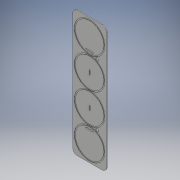
# Autodesk Inventor part: Cewki_840
Saved by Autodesk Inventor 2017 (Build 210142000, 142)
## iProperties
Created: 2019-10-27
Part Number: Cewki_840
Material: Ogólny
Document SubType Name: Modeling
Designer: patry
Density: 1 g/cm^3
Appearance: Domyślna
Author: patry
Autodesk Inventor part; units mm, degrees
ref_plane "YZ Plane" through (0, 0, 0) normal (1, 0, 0) x (0, 1, 0)
ref_plane "XZ Plane" through (0, 0, 0) normal (0, 1, 0) x (-1, 0, 0)
ref_plane "XY Plane" through (0, 0, 0) normal (0, 0, 1) x (1, 0, 0)
sketch "Szkic1" plane through (0, 0, 0) normal (0, 1, 0) x (-1, 0, 0)
  line L0 (-112.5, 420) -> (112.5, 420)
  line L1 (112.5, 420) -> (112.5, 262)
  line L2 (112.5, -420) -> (-112.5, -420)
  line L3 (-112.5, -420) -> (-112.5, 27)
  line L4 (-112.5, 420) -> (112.5, -420) construction
  line L5 (112.5, 420) -> (-112.5, -420) construction
  circle A0 centre (0, -307.5) radius 102.5
  circle A1 centre (0, -307.5) radius 95
  circle A2 centre (0, -102.5) radius 102.5
  circle A3 centre (0, -102.5) radius 95
  circle A4 centre (0, 102.5) radius 102.5
  circle A5 centre (0, 102.5) radius 95
  circle A6 centre (0, 307.5) radius 102.5
  circle A7 centre (0, 307.5) radius 95
  line L6 (-112.5, 27) -> (-112.5, 420)
  line L7 (0, 420) -> (0, -420) construction
  line L8 (112.5, 262) -> (112.5, 257)
  line L9 (112.5, 257) -> (112.5, -193)
  line L10 (112.5, -197.6604) -> (112.5, -420)
  line L11 (112.5, -193) -> (112.5, -197.6604)
  line L12 (-182, -225) -> (183, -225) construction
  line L13 (-175, 225) -> (225, 225) construction
  line L14 (-221, -230.5) -> (174, -230.5) construction
  line L15 (-175, 230.5) -> (202.5, 230.5) construction
  line L16 (23, 225) -> (-23, 225)
  line L17 (-25, 227) -> (-25, 228.5)
  line L18 (-23, 230.5) -> (23, 230.5)
  line L19 (25, 228.5) -> (25, 227)
  line L20 (-226, 0) -> (183, 0) construction
  arc A8 (23, 225) -> (25, 227) centre (23, 227) ccw
  arc A9 (25, 228.5) -> (23, 230.5) centre (23, 228.5) ccw
  arc A10 (-25, 227) -> (-23, 225) centre (-23, 227) ccw
  arc A11 (-23, 230.5) -> (-25, 228.5) centre (-23, 228.5) ccw
  line L21 (23, -225) -> (-23, -225)
  line L22 (-25, -227) -> (-25, -228.5)
  line L23 (-23, -230.5) -> (23, -230.5)
  line L24 (25, -228.5) -> (25, -227)
  arc A12 (25, -227) -> (23, -225) centre (23, -227) ccw
  arc A13 (23, -230.5) -> (25, -228.5) centre (23, -228.5) ccw
  arc A14 (-23, -225) -> (-25, -227) centre (-23, -227) ccw
  arc A15 (-25, -228.5) -> (-23, -230.5) centre (-23, -228.5) ccw
  line L25 (0, -212.5) -> (0, 284.5) construction
  line L26 (-55, -249) -> (-55, 249) construction
  line L27 (-0.75, -87.5) -> (0.75, -87.5)
  line L28 (2.75, -89.5) -> (2.75, -115.5)
  line L29 (0.75, -117.5) -> (-0.75, -117.5)
  line L30 (-2.75, -115.5) -> (-2.75, -89.5)
  line L31 (-2.75, -87.5) -> (2.75, -117.5) construction
  line L32 (2.75, -87.5) -> (-2.75, -117.5) construction
  line L33 (-0.75, 87.5) -> (0.75, 87.5)
  line L34 (2.75, 89.5) -> (2.75, 115.5)
  line L35 (0.75, 117.5) -> (-0.75, 117.5)
  line L36 (-2.75, 115.5) -> (-2.75, 89.5)
  line L37 (-2.75, 87.5) -> (2.75, 117.5) construction
  line L38 (2.75, 87.5) -> (-2.75, 117.5) construction
  arc A16 (2.75, 115.5) -> (0.75, 117.5) centre (0.75, 115.5) ccw
  arc A17 (-0.75, 117.5) -> (-2.75, 115.5) centre (-0.75, 115.5) ccw
  arc A18 (-2.75, 89.5) -> (-0.75, 87.5) centre (-0.75, 89.5) ccw
  arc A19 (0.75, 87.5) -> (2.75, 89.5) centre (0.75, 89.5) ccw
  arc A20 (0.75, -117.5) -> (2.75, -115.5) centre (0.75, -115.5) ccw
  arc A21 (2.75, -89.5) -> (0.75, -87.5) centre (0.75, -89.5) ccw
  arc A22 (-0.75, -87.5) -> (-2.75, -89.5) centre (-0.75, -89.5) ccw
  arc A23 (-2.75, -115.5) -> (-0.75, -117.5) centre (-0.75, -115.5) ccw
  circle A24 centre (-51.25, 205) radius 10
  circle A25 centre (-51.25, -205) radius 10
  point P0 (0, 0)
  point P1 (98, -242)
  point P2 (25, 225)
  point P3 (-25, 230.5)
  point P4 (-25, 225)
  point P5 (25, 230.5)
  point P6 (25, -225)
  point P7 (-25, -230.5)
  point P8 (-25, -225)
  point P9 (25, -230.5)
  point P10 (-86.6642, -225)
  point P11 (0, -102.5)
  point P12 (0, 102.5)
  point P13 (0, 102.5)
  point P14 (0, -102.5)
  point P15 (0, 102.5)
  dimension "d0" = 225
  dimension "d1" = 840
  dimension "d2" = 112.5
  dimension "d3" = 205
  dimension "d4" = 205
  dimension "d5" = 205
  dimension "d6" = 102.5
  dimension "d7" = 205
  dimension "d8" = 190
  dimension "d9" = 205
  dimension "d10" = 190
  dimension "d13" = 205
  dimension "d14" = 190
  dimension "d17" = 205
  dimension "d18" = 190
  dimension "d57" = 450
  dimension "d58" = 5.5
  dimension "d59" = 5.5
  dimension "d60" = 225
  dimension "d65" = 50
  dimension "d67" = 2
  dimension "d68" = 2
  dimension "d72" = 25
  dimension "d74" = 5.5
  dimension "d75" = 30
  dimension "d78" = 5.5
  dimension "d79" = 30
  dimension "d82" = 205
  dimension "d103" = 2
  dimension "d104" = 2
  dimension "d105" = 2
  dimension "d106" = 2
  dimension "d107" = 2
  dimension "d108" = 2
  dimension "d109" = 2
  dimension "d110" = 102.5
  dimension "d111" = 102.5
  dimension "d112" = 51.25
  dimension "d113" = 20
  dimension "d114" = 20
  constraints: 78 end point, 35 point on line, 32 point on circle, 26 centre point, 24 tangent, 17 parallel, 16 symmetric about line, 12 midpoint, 11 coincident, 8 horizontal, 8 perpendicular, 4 vertical alignment, 3 equal radius, 2 vertical, 1 collinear, 4 other
  measures "d0" distance of L2.start L2.end
  measures "d1" distance of L0.end L2.start
  measures "d2" distance from line of L1 point (0, 307.5)
  measures "d3" distance of point (0, 102.5) point (0, 307.5)
  measures "d4" distance of point (0, 102.5) point (0, -102.5)
  measures "d5" distance of point (0, -102.5) point (0, -307.5)
  measures "d6" distance of point (0, 0) point (0, 102.5)
  measures "d7" diameter of A0
  measures "d8" diameter of A1
  measures "d9" diameter of A2
  measures "d10" diameter of A3
  measures "d13" diameter of A4
  measures "d14" diameter of A5
  measures "d17" diameter of A6
  measures "d18" diameter of A7
  measures "d57" distance between parallel lines of L12 L13
  measures "d58" distance between parallel lines of L15 L13
  measures "d59" distance between parallel lines of L12 L14
  measures "d60" distance from line of point (0, 0) L12
  measures "d65" distance between parallel lines of L19 L17
  measures "d67" radius of A8
  measures "d68" radius of A11
  measures "d72" distance from line of L19.end L25
  measures "d74" distance of L31.end L32.end
  measures "d75" distance of L32.start L31.end
  measures "d78" distance of L38.end L37.end
  measures "d79" distance of L37.end L38.start
  measures "d82" distance of point (0, 102.5) point (0, -102.5)
  measures "d103" radius of A17
  measures "d104" radius of A16
  measures "d105" radius of A18
  measures "d106" radius of A19
  measures "d107" radius of A22
  measures "d108" radius of A21
  measures "d109" radius of A20
  measures "d110" vertical distance of point (0, -102.5) point (-51.25, -205)
  measures "d111" vertical distance of point (0, 102.5) point (-51.25, 205)
  measures "d112" horizontal distance of point (0, 307.5) point (-51.25, 205)
  measures "d113" diameter of A24
  measures "d114" diameter of A25
extrude "Wyciągnięcie proste1" add sketch "Szkic1" along normal blind 5 contours L0 L1 L8 L9 L11 L10 L2 L3 L6 | A0 | A6 | A4 | A2 | A1 | A3 | A5 | A7
extrude "Wyciągnięcie proste2" cut sketch "Szkic1" along normal blind 2 contours A0 | A6 | A4 | A2
fillet "Zaokrąglenie1" radius 30 4 edges at (112.5, 2.5, -420) (-112.5, 2.5, -420) (-112.5, 2.5, 420) (112.5, 2.5, 420)
extrude "Wyciągnięcie proste3" cut sketch "Szkic1" along normal blind 10 contours A24 | A25
equation "\"d0\" = sred_zew + odsuniecie"
equation "\"d1\" = 3 * odl_cewkii + sred_zew + odsuniecie"
equation "\"d2\" = 0.5 * d0"
equation "\"d3\" = d5"
equation "\"d4\" = d5"
equation "\"d5\" = odl_cewkii"
equation "\"d6\" = 0.5 * d4"
equation "\"d7\" = sred_zew"
equation "\"d8\" = sred_wew"
equation "\"d9\" = d11"
equation "\"d10\" = d12"
equation "\"d13\" = d15"
equation "\"d14\" = d16"
equation "\"d17\" = d19"
equation "\"d18\" = d20"
equation "\"odl_cewkii\" = 205"
equation "\"sred_wew\" = 190"
equation "\"sred_zew\" = 205"
equation "\"odsuniecie\" = 20"
equation "\"d11\" = 205"
equation "\"d12\" = 190"
equation "\"d15\" = 205"
equation "\"d16\" = 190"
equation "\"d19\" = 205"
equation "\"d20\" = 190"
